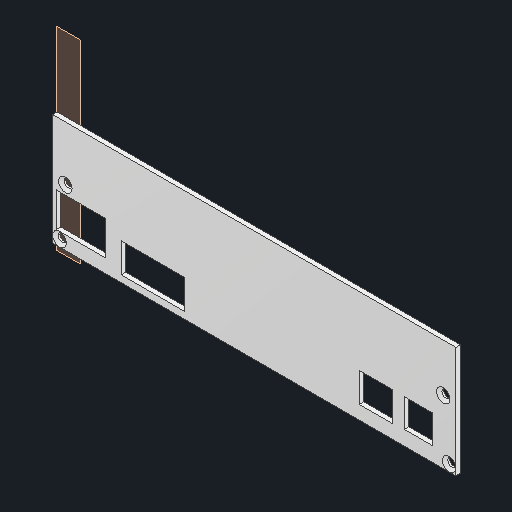
# Autodesk Inventor part: ceil_front
Saved by Autodesk Inventor 2023 (Build 270158000, 158)
## iProperties
Created: 2024-04-28
Part Number: ceil_front
Material: ABS Plastic
Document SubType Name: Modeling
Designer: szymo
Density: 1.06 g/cm^3
Appearance: Smooth - White
Mass: 16.2132 g
Surface Area: 168.318 cm^2
Volume: 15.2955 cm^3
Author: szymo
Autodesk Inventor part; units mm, degrees
ref_plane "YZ Plane" through (0, 0, 0) normal (1, 0, 0) x (0, 1, 0)
ref_plane "XZ Plane" through (0, 0, 0) normal (0, 1, 0) x (-1, 0, 0)
ref_plane "XY Plane" through (0, 0, 0) normal (0, 0, 1) x (1, 0, 0)
ref_plane "Work Plane1" through (0, 0, 0) normal (0, 0, 1) x (1, 0, 0)
sketch "Sketch1" plane through (0, 0, 0) normal (0, 0, 1) x (1, 0, 0)
  circle A0 centre (118.7, -21.5445) radius 2.5 projected
  circle A1 centre (113.95, -8.8843) radius 2.5 projected
  circle A2 centre (64.05, -19.8657) radius 2.5 projected
  circle A3 centre (59.3, -7.2055) radius 2.5 projected
  circle A4 centre (64.05, -8.8843) radius 2.5 projected
  circle A5 centre (59.3, -21.5445) radius 2.5 projected
  circle A6 centre (118.7, -7.2055) radius 2.5 projected
  circle A7 centre (113.95, -19.8657) radius 2.5 projected
  line L0 (84.5, 12.4325) -> (84.5, -11.5675) projected
  line L1 (84.5, -11.5675) -> (72.5, -11.5675) projected
  line L2 (72.5, -11.5675) -> (72.5, 4.5875) projected
  circle A8 centre (69.5, 4.5875) radius 3 projected
  line L3 (72.5, 4.5875) -> (72.5, 12.4325) projected
  line L4 (72.5, 12.4325) -> (84.5, 12.4325) projected
  arc A9 (105.5, 4.2836) -> (105.5, 4.8914) centre (108.4846, 4.5875) ccw projected
  line L5 (105.5, 4.2836) -> (105.5, -11.5675) projected
  line L6 (105.5, -11.5675) -> (93.5, -11.5675) projected
  line L7 (93.5, -11.5675) -> (93.5, 12.4325) projected
  line L8 (93.5, 12.4325) -> (105.5, 12.4325) projected
  line L9 (105.5, 12.4325) -> (105.5, 4.8914) projected
  circle A10 centre (108.4462, 27.5) radius 3 projected
  circle A11 centre (69.5, 27.5) radius 3 projected
  circle A12 centre (89, 0.9661) radius 3 projected
  circle A13 centre (89, 29.5) radius 3 projected
  arc A14 (175, 0) -> (178, -3) centre (175, -3) ccw projected
  line L10 (175, 0) -> (112.5, 0) projected
  line L11 (112.5, 0) -> (112.5, 55) projected
  line L12 (112.5, 55) -> (65.5, 55) projected
  line L13 (65.5, 55) -> (65.5, 0) projected
  line L14 (65.5, 0) -> (3, 0) projected
  arc A15 (0, -3) -> (3, 0) centre (3, -3) ccw projected
  line L15 (0, -3) -> (0, -25.75) projected
  arc A16 (3, -28.75) -> (0, -25.75) centre (3, -25.75) ccw projected
  line L16 (3, -28.75) -> (175, -28.75) projected
  arc A17 (178, -25.75) -> (175, -28.75) centre (175, -25.75) ccw projected
  line L17 (178, -25.75) -> (178, -3) projected
  circle A18 centre (3, -25.75) radius 2.3 projected
  circle A19 centre (3, -3) radius 2.3 projected
  circle A20 centre (3, -74.8889) radius 2.3 projected
  line L18 (0, 0) -> (6, 0) projected
  line L19 (0, -77.8889) -> (0, 0) projected
  line L20 (0, -77.8889) -> (6, -77.8889) projected
  line L21 (6, -71.8889) -> (6, -77.8889) projected
  line L22 (6, -71.8889) -> (1.6, -71.8889) projected
  line L23 (1.6, -71.8889) -> (1.6, -56.7889) projected
  line L24 (1.6, -56.7889) -> (9.6, -56.7889) projected
  line L25 (9.6, -44.7889) -> (9.6, -56.7889) projected
  line L26 (3, -44.7889) -> (9.6, -44.7889) projected
  line L27 (3, -28.75) -> (3, -44.7889) projected
  line L28 (3, -28.75) -> (6, -28.75) projected
  line L29 (6, -28.75) -> (6, -22.75) projected
  line L30 (6, -22.75) -> (3, -22.75) projected
  line L31 (3, -6) -> (3, -22.75) projected
  line L32 (3, -6) -> (6, -6) projected
  line L33 (6, -6) -> (6, 0) projected
  circle A21 centre (5.6, -52.7889) radius 2.6 projected
  circle A22 centre (175, -3) radius 2.3 projected
  circle A23 centre (175, -25.75) radius 2.3 projected
  line L34 (175, -28.75) -> (175, -41.8889) projected
  line L35 (168.4, -41.8889) -> (175, -41.8889) projected
  line L36 (168.4, -53.8889) -> (168.4, -41.8889) projected
  line L37 (175, -53.8889) -> (168.4, -53.8889) projected
  line L38 (175, -53.8889) -> (175, -71.8889) projected
  line L39 (175, -71.8889) -> (172, -71.8889) projected
  line L40 (172, -71.8889) -> (172, -77.8889) projected
  line L41 (178, -77.8889) -> (172, -77.8889) projected
  line L42 (178, -77.8889) -> (178, 0) projected
  line L43 (178, 0) -> (172, 0) projected
  line L44 (172, 0) -> (172, -6) projected
  line L45 (172, -6) -> (175, -6) projected
  line L46 (175, -6) -> (175, -22.75) projected
  line L47 (175, -22.75) -> (172, -22.75) projected
  line L48 (172, -22.75) -> (172, -28.75) projected
  line L49 (172, -28.75) -> (175, -28.75) projected
  circle A24 centre (175, -74.8889) radius 2.3 projected
  circle A25 centre (172.4, -49.8889) radius 2.6 projected
  line L50 (156.2, -70.4889) -> (156.2, -59.9889) projected
  line L51 (166.7, -59.9889) -> (156.2, -59.9889) projected
  line L52 (166.7, -59.9889) -> (166.7, -70.4889) projected
  line L53 (156.2, -70.4889) -> (166.7, -70.4889) projected
  line L54 (149, -59.8889) -> (149, -70.8889) projected
  line L55 (149, -70.8889) -> (136.35, -70.8889) projected
  line L56 (136.35, -70.8889) -> (136.35, -59.8889) projected
  line L57 (136.35, -59.8889) -> (149, -59.8889) projected
  line L58 (135, -53.8889) -> (135, -71.8889) projected
  line L59 (135, -71.8889) -> (175, -71.8889) projected
  line L60 (175, -71.8889) -> (175, -53.8889) projected
  line L61 (175, -53.8889) -> (135, -53.8889) projected
  circle A26 centre (137.85, -56.7389) radius 1.5 projected
  circle A27 centre (172.15, -56.7389) radius 1.5 projected
  line L62 (31.25, -62.8889) -> (31.25, -73.8889) projected
  line L63 (31.25, -73.8889) -> (57.25, -73.8889) projected
  line L64 (57.25, -73.8889) -> (57.25, -62.8889) projected
  line L65 (57.25, -62.8889) -> (31.25, -62.8889) projected
  line L66 (9.6, -56.7889) -> (23.3, -56.7889) projected
  line L67 (23.3, -56.7889) -> (23.3, -59.8889) projected
  line L68 (23.3, -59.8889) -> (23.3, -65.1889) projected
  line L69 (3, -71.8889) -> (23.3, -71.8889) projected
  line L70 (23.3, -61.8889) -> (23.3, -74.8889) projected
  line L71 (30.25, -61.8889) -> (30.25, -74.8889)
  line L72 (30.25, -74.8889) -> (58.25, -74.8889)
  line L73 (58.25, -74.8889) -> (58.25, -61.8889)
  line L74 (58.25, -61.8889) -> (30.25, -61.8889)
  line L75 (150, -58.8889) -> (150, -71.8889)
  line L76 (150, -71.8889) -> (135.35, -71.8889)
  line L77 (135.35, -71.8889) -> (135.35, -58.8889)
  line L78 (135.35, -58.8889) -> (150, -58.8889)
  line L79 (155.2, -58.9889) -> (155.2, -71.4889)
  line L80 (155.2, -71.4889) -> (167.7, -71.4889)
  line L81 (167.7, -71.4889) -> (167.7, -58.9889)
  line L82 (167.7, -58.9889) -> (155.2, -58.9889)
  line L83 (0, -28.75) -> (178, -28.75)
  line L84 (178, -28.75) -> (178, -77.8889)
  line L85 (178, -77.8889) -> (0, -77.8889)
  line L86 (0, -77.8889) -> (0, -28.75)
  line L87 (147.9, -18.975) -> (147.9, -9.775) projected
  spline S0 degree 3 poles (147.9, -9.775) (147.9, -9.6319) (147.9163, -9.3812) (147.9666, -9.0958) (148.0181, -8.8833) (148.0595, -8.7423) (148.12, -8.5679) (148.1761, -8.4292) (148.2544, -8.2606) (148.3231, -8.1302) (148.416, -7.9727) (148.4957, -7.8511) (148.6018, -7.7049) (148.6917, -7.5925) (148.8338, -7.4311) (148.985, -7.2799) (149.2059, -7.0923) (149.3854, -6.9628) (149.5759, -6.8435) (149.7083, -6.7693) (149.8633, -6.6924) (149.97, -6.6451) (150.0794, -6.6013) (150.1527, -6.5741) (150.2632, -6.5365) (150.3745, -6.5028) (150.58, -6.4499) (150.8061, -6.4076) (151.1474, -6.3724) (151.4526, -6.3724) (151.7939, -6.4076) (152.02, -6.4499) (152.2255, -6.5028) (152.3368, -6.5365) (152.4473, -6.5741) (152.5206, -6.6013) (152.63, -6.6451) (152.7367, -6.6924) (152.8917, -6.7693) (153.0241, -6.8435) (153.2146, -6.9628) (153.3941, -7.0923) (153.615, -7.2799) (153.7662, -7.4311) (153.9083, -7.5925) (153.9982, -7.7049) (154.1043, -7.8511) (154.184, -7.9727) (154.2769, -8.1302) (154.3456, -8.2606) (154.4239, -8.4292) (154.48, -8.5679) (154.5405, -8.7423) (154.5819, -8.8833) (154.6334, -9.0958) (154.6837, -9.3812) (154.7, -9.6319) (154.7, -9.775) knots -0.380025 -0.380025 -0.380025 -0.380025 -0.348357 -0.324605 -0.316688 -0.300853 -0.292936 -0.277102 -0.269185 -0.25335 -0.245433 -0.229599 -0.221682 -0.205847 -0.19793 -0.174178 -0.158344 -0.134592 -0.126675 -0.110841 -0.102924 -0.091048 -0.087089 -0.079172 -0.075213 -0.063338 -0.05542 -0.031669 -0.015834 0.015834 0.031669 0.05542 0.063338 0.075213 0.079172 0.087089 0.091048 0.102924 0.110841 0.126675 0.134592 0.158344 0.174178 0.19793 0.205847 0.221682 0.229599 0.245433 0.25335 0.269185 0.277102 0.292936 0.300853 0.316688 0.324605 0.348357 0.380025 0.380025 0.380025 0.380025 projected
  line L88 (154.7, -9.775) -> (154.7, -18.975) projected
  spline S1 degree 3 poles (154.7, -18.975) (154.7, -19.1181) (154.6837, -19.3688) (154.6334, -19.6542) (154.5819, -19.8667) (154.5405, -20.0077) (154.48, -20.1821) (154.4239, -20.3208) (154.3456, -20.4894) (154.2769, -20.6198) (154.184, -20.7773) (154.1043, -20.8989) (153.9982, -21.0451) (153.9083, -21.1575) (153.7662, -21.3189) (153.615, -21.4701) (153.3941, -21.6577) (153.2146, -21.7872) (153.0241, -21.9065) (152.8917, -21.9807) (152.7367, -22.0576) (152.63, -22.1049) (152.5206, -22.1487) (152.4473, -22.1759) (152.3368, -22.2135) (152.2255, -22.2472) (152.02, -22.3001) (151.7939, -22.3424) (151.4526, -22.3776) (151.1474, -22.3776) (150.8061, -22.3424) (150.58, -22.3001) (150.3745, -22.2472) (150.2632, -22.2135) (150.1527, -22.1759) (150.0794, -22.1487) (149.97, -22.1049) (149.8633, -22.0576) (149.7083, -21.9807) (149.5759, -21.9065) (149.3854, -21.7872) (149.2059, -21.6577) (148.985, -21.4701) (148.8338, -21.3189) (148.6917, -21.1575) (148.6018, -21.0451) (148.4957, -20.8989) (148.416, -20.7773) (148.3231, -20.6198) (148.2544, -20.4894) (148.1761, -20.3208) (148.12, -20.1821) (148.0595, -20.0077) (148.0181, -19.8667) (147.9666, -19.6542) (147.9163, -19.3688) (147.9, -19.1181) (147.9, -18.975) knots 0.368505 0.368505 0.368505 0.368505 0.400174 0.423925 0.431842 0.447677 0.455594 0.471428 0.479345 0.49518 0.503097 0.518931 0.526849 0.542683 0.5506 0.574352 0.590186 0.613938 0.621855 0.637689 0.645607 0.657482 0.661441 0.669358 0.673317 0.685193 0.69311 0.716861 0.732696 0.764365 0.780199 0.803951 0.811868 0.823744 0.827702 0.835619 0.839578 0.851454 0.859371 0.875205 0.883123 0.906874 0.922709 0.94646 0.954377 0.970212 0.978129 0.993963 1.00188 1.017715 1.025632 1.041466 1.049384 1.065218 1.073135 1.096887 1.128556 1.128556 1.128556 1.128556 projected
  spline S2 degree 3 poles (30.1, -18.975) (30.1, -19.1181) (30.0837, -19.3688) (30.0334, -19.6542) (29.9819, -19.8667) (29.9405, -20.0077) (29.88, -20.1821) (29.8239, -20.3208) (29.7456, -20.4894) (29.6769, -20.6198) (29.584, -20.7773) (29.5043, -20.8989) (29.3982, -21.0451) (29.3083, -21.1575) (29.1662, -21.3189) (29.015, -21.4701) (28.7941, -21.6577) (28.6146, -21.7872) (28.4241, -21.9065) (28.2917, -21.9807) (28.1367, -22.0576) (28.03, -22.1049) (27.9206, -22.1487) (27.8473, -22.1759) (27.7368, -22.2135) (27.6255, -22.2472) (27.42, -22.3001) (27.1939, -22.3424) (26.8526, -22.3776) (26.5474, -22.3776) (26.2061, -22.3424) (25.98, -22.3001) (25.7745, -22.2472) (25.6632, -22.2135) (25.5527, -22.1759) (25.4794, -22.1487) (25.37, -22.1049) (25.2633, -22.0576) (25.1083, -21.9807) (24.9759, -21.9065) (24.7854, -21.7872) (24.6059, -21.6577) (24.385, -21.4701) (24.2338, -21.3189) (24.0917, -21.1575) (24.0018, -21.0451) (23.8957, -20.8989) (23.816, -20.7773) (23.7231, -20.6198) (23.6544, -20.4894) (23.5761, -20.3208) (23.52, -20.1821) (23.4595, -20.0077) (23.4181, -19.8667) (23.3666, -19.6542) (23.3163, -19.3688) (23.3, -19.1181) (23.3, -18.975) knots 0.368505 0.368505 0.368505 0.368505 0.400174 0.423925 0.431842 0.447677 0.455594 0.471428 0.479345 0.49518 0.503097 0.518931 0.526849 0.542683 0.5506 0.574352 0.590186 0.613938 0.621855 0.637689 0.645607 0.657482 0.661441 0.669358 0.673317 0.685193 0.69311 0.716861 0.732696 0.764365 0.780199 0.803951 0.811868 0.823744 0.827702 0.835619 0.839578 0.851454 0.859371 0.875205 0.883123 0.906874 0.922709 0.94646 0.954377 0.970212 0.978129 0.993963 1.00188 1.017715 1.025632 1.041466 1.049384 1.065218 1.073135 1.096887 1.128556 1.128556 1.128556 1.128556 projected
  line L89 (23.3, -18.975) -> (23.3, -9.775) projected
  spline S3 degree 3 poles (23.3, -9.775) (23.3, -9.6319) (23.3163, -9.3812) (23.3666, -9.0958) (23.4181, -8.8833) (23.4595, -8.7423) (23.52, -8.5679) (23.5761, -8.4292) (23.6544, -8.2606) (23.7231, -8.1302) (23.816, -7.9727) (23.8957, -7.8511) (24.0018, -7.7049) (24.0917, -7.5925) (24.2338, -7.4311) (24.385, -7.2799) (24.6059, -7.0923) (24.7854, -6.9628) (24.9759, -6.8435) (25.1083, -6.7693) (25.2633, -6.6924) (25.37, -6.6451) (25.4794, -6.6013) (25.5527, -6.5741) (25.6632, -6.5365) (25.7745, -6.5028) (25.98, -6.4499) (26.2061, -6.4076) (26.5474, -6.3724) (26.8526, -6.3724) (27.1939, -6.4076) (27.42, -6.4499) (27.6255, -6.5028) (27.7368, -6.5365) (27.8473, -6.5741) (27.9206, -6.6013) (28.03, -6.6451) (28.1367, -6.6924) (28.2917, -6.7693) (28.4241, -6.8435) (28.6146, -6.9628) (28.7941, -7.0923) (29.015, -7.2799) (29.1662, -7.4311) (29.3083, -7.5925) (29.3982, -7.7049) (29.5043, -7.8511) (29.584, -7.9727) (29.6769, -8.1302) (29.7456, -8.2606) (29.8239, -8.4292) (29.88, -8.5679) (29.9405, -8.7423) (29.9819, -8.8833) (30.0334, -9.0958) (30.0837, -9.3812) (30.1, -9.6319) (30.1, -9.775) knots -0.380025 -0.380025 -0.380025 -0.380025 -0.348357 -0.324605 -0.316688 -0.300853 -0.292936 -0.277102 -0.269185 -0.25335 -0.245433 -0.229599 -0.221682 -0.205847 -0.19793 -0.174178 -0.158344 -0.134592 -0.126675 -0.110841 -0.102924 -0.091048 -0.087089 -0.079172 -0.075213 -0.063338 -0.05542 -0.031669 -0.015834 0.015834 0.031669 0.05542 0.063338 0.075213 0.079172 0.087089 0.091048 0.102924 0.110841 0.126675 0.134592 0.158344 0.174178 0.19793 0.205847 0.221682 0.229599 0.245433 0.25335 0.269185 0.277102 0.292936 0.300853 0.316688 0.324605 0.348357 0.380025 0.380025 0.380025 0.380025 projected
  line L90 (30.1, -9.775) -> (30.1, -18.975) projected
  point P0 (3, -28.75)
  point P1 (175, -28.75)
  point P2 (135.35, -71.8889)
  dimension "d0" = 1
  dimension "d1" = 1
  dimension "d2" = 1
  constraints: 32 end point, 2 parallel, 1 horizontal, 1 horizontal alignment, 1 perpendicular, 1 point on line, 9 other
  measures "d0" distance between parallel lines of L65 L74
  measures "d1" distance between parallel lines of L57 L78
  measures "d2" distance between parallel lines of L51 L82
extrude "Extrusion1" add sketch "Sketch1" along normal blind 2 contours L42 L41 L40 L39 L38 L37 L36 L35 L34 L83 | L34 L35 L36 L61 L58 L59 L40 L85 L21 L69 L70 L68 L67 L66 L25 L26 L27 L16 | L27 L26 L25 L24 L23 L22 L21 L20 L19 L83 | L59 L75 L78 L77 L58 L61 L37 L38 L39 | A20 | A21 | A24 | A25 | A26 | A27
sketch "Sketch2" plane through (0, 0, 2) normal (0, 0, 1) x (1, 0, 0)
  circle A0 centre (3, -25.75) radius 2.3 projected
  circle A1 centre (3, -3) radius 2.3 projected
  circle A2 centre (3, -74.8889) radius 2.3 projected
  line L0 (0, 0) -> (6, 0) projected
  line L1 (0, -77.8889) -> (0, 0) projected
  line L2 (0, -77.8889) -> (6, -77.8889) projected
  line L3 (6, -71.8889) -> (6, -77.8889) projected
  line L4 (6, -71.8889) -> (1.6, -71.8889) projected
  line L5 (1.6, -71.8889) -> (1.6, -56.7889) projected
  line L6 (1.6, -56.7889) -> (9.6, -56.7889) projected
  line L7 (9.6, -44.7889) -> (9.6, -56.7889) projected
  line L8 (3, -44.7889) -> (9.6, -44.7889) projected
  line L9 (3, -28.75) -> (3, -44.7889) projected
  line L10 (3, -28.75) -> (6, -28.75) projected
  line L11 (6, -28.75) -> (6, -22.75) projected
  line L12 (6, -22.75) -> (3, -22.75) projected
  line L13 (3, -6) -> (3, -22.75) projected
  line L14 (3, -6) -> (6, -6) projected
  line L15 (6, -6) -> (6, 0) projected
  circle A3 centre (5.6, -52.7889) radius 2.6 projected
  circle A4 centre (172.4, -49.8889) radius 2.6 projected
  circle A5 centre (175, -3) radius 2.3 projected
  circle A6 centre (175, -25.75) radius 2.3 projected
  line L16 (175, -28.75) -> (175, -41.8889) projected
  line L17 (168.4, -41.8889) -> (175, -41.8889) projected
  line L18 (168.4, -53.8889) -> (168.4, -41.8889) projected
  line L19 (175, -53.8889) -> (168.4, -53.8889) projected
  line L20 (175, -53.8889) -> (175, -71.8889) projected
  line L21 (175, -71.8889) -> (172, -71.8889) projected
  line L22 (172, -71.8889) -> (172, -77.8889) projected
  line L23 (178, -77.8889) -> (172, -77.8889) projected
  line L24 (178, -77.8889) -> (178, 0) projected
  line L25 (178, 0) -> (172, 0) projected
  line L26 (172, 0) -> (172, -6) projected
  line L27 (172, -6) -> (175, -6) projected
  line L28 (175, -6) -> (175, -22.75) projected
  line L29 (175, -22.75) -> (172, -22.75) projected
  line L30 (172, -22.75) -> (172, -28.75) projected
  line L31 (172, -28.75) -> (175, -28.75) projected
  circle A7 centre (175, -74.8889) radius 2.3 projected
  circle A8 centre (172.4, -49.8889) radius 2.6 projected
  constraints: 4 coincident
hole "Hole1" at (5.6, -52.7889, 2) at (3, -74.8889, 2) at (175, -74.8889, 2) at (172.4, -49.8889, 2) direction (0, 0, -1) diameter 3.6 end through all countersink diameter 6 countersink angle 90 clearance for "Countersunk Flat Head Screw ISO 2009/7046" size "M3" standard "ISO"
body "Solid1"
